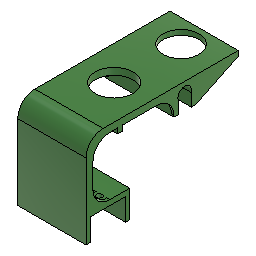
5_Assembly_Support Bat v5 (Autodesk Fusion 360 archive; units mm, degrees)
design "Support Button"
Autodesk Fusion 360 part; units mm, degrees
sketch "Sketch2" plane through (0, 0, 0) normal (1, 0, 0) x (0, 1, 0) in component "Support Batt"
  circle A0 centre (154.2359, 79.3135) radius 4
  line L0 (99.2359, 44.7135) -> (119.2359, 44.7135)
  line L1 (119.2359, 31.7135) -> (119.2359, 44.7135)
  line L2 (99.2359, 31.7135) -> (99.2359, 44.7135)
  line L3 (160.5859, 85.8135) -> (106.4359, 85.8135)
  line L4 (50.5431, 31.7135) -> (52.3447, 31.7135)
  line L5 (52.3447, 31.7135) -> (217.041, 31.7135) construction
  line L6 (96.4359, 75.8135) -> (96.4359, 31.7135)
  line L7 (96.4359, 31.7135) -> (98.9359, 31.7135)
  line L8 (98.9359, 44.7135) -> (119.5359, 44.7135)
  line L9 (119.5359, 44.7135) -> (119.5359, 31.7135)
  line L10 (98.9359, 44.7135) -> (98.9359, 31.7135)
  line L11 (119.5359, 31.7135) -> (122.0359, 31.7135)
  line L12 (154.2359, 83.3135) -> (160.5859, 83.3135) construction
  line L13 (160.5859, 85.8135) -> (160.5859, 70.8135)
  line L14 (158.0859, 70.8135) -> (160.5859, 70.8135)
  line L15 (158.0859, 78.2283) -> (158.0859, 70.8135)
  line L16 (150.3859, 78.2283) -> (150.3859, 70.8135)
  line L17 (150.3859, 70.8135) -> (147.8859, 70.8135)
  line L18 (150.3859, 70.8135) -> (158.0859, 70.8135) construction
  line L19 (154.2359, 79.3135) -> (154.2359, 70.8135) construction
  line L20 (147.8859, 70.8135) -> (147.8859, 71.8135)
  line L21 (137.8859, 81.8135) -> (110.4359, 81.8135)
  line L22 (122.0359, 31.7135) -> (122.0359, 47.7135)
  line L23 (122.0359, 47.7135) -> (110.4359, 47.7135)
  line L24 (100.4359, 57.7135) -> (100.4359, 71.8135)
  arc A1 (110.4359, 81.8135) -> (100.4359, 71.8135) centre (110.4359, 71.8135) ccw
  arc A2 (147.8859, 71.8135) -> (137.8859, 81.8135) centre (137.8859, 71.8135) ccw
  arc A3 (100.4359, 57.7135) -> (110.4359, 47.7135) centre (110.4359, 57.7135) ccw
  arc A4 (158.0859, 78.2283) -> (150.3859, 78.2283) centre (154.2359, 79.3135) ccw
  arc A5 (106.4359, 85.8135) -> (96.4359, 75.8135) centre (106.4359, 75.8135) ccw
  line L25 (114.8859, 81.8135) -> (117.8859, 81.8135)
  line L26 (117.8859, 81.8135) -> (117.8859, 78.8135)
  line L27 (117.8859, 78.8135) -> (114.8859, 78.8135)
  line L28 (114.8859, 78.8135) -> (114.8859, 81.8135)
  line L29 (160.5859, 85.8135) -> (185.5859, 85.8135)
  line L30 (185.5859, 85.8135) -> (185.5859, 82.8135)
  line L31 (185.5859, 82.8135) -> (160.5859, 82.8135)
  line L32 (160.5859, 82.8135) -> (160.5859, 85.8135)
  line L33 (160.5859, 70.8135) -> (185.5859, 82.8135)
  point P0 (96.4359, 85.8135)
  point P1 (100.4359, 81.8135)
  dimension "d2" = 0.3
  dimension "d3" = 0.3
  dimension "d4" = 2.5
  dimension "d5" = 2.5
  dimension "d6" = 2.5
  dimension "d7" = 2.5
  dimension "d8" = 8
  dimension "d9" = 15
  dimension "d10" = 7.7
  dimension "d11" = 2.5
  dimension "d12" = 4
  dimension "d13" = 4
  dimension "d14" = 3
  dimension "d15" = 10
  dimension "d68" = 10
  dimension "d69" = 3
  dimension "d70" = 3
  dimension "d71" = 30
  dimension "d80" = 25
  dimension "d81" = 3
  constraint horizontal L3
  constraint horizontal L4
  constraint parallel L4 L5
  constraint coincident L2.start L5
  constraint coincident L5 L6.end
  constraint perpendicular L5 L6
  constraint coincident L5 L7.end
  constraint perpendicular L6 L8
  constraint coincident L5 L9.end
  constraint perpendicular L8 L9
  constraint perpendicular L7 L10
  constraint coincident L0.start L8
  constraint coincident L5 L11.end
  constraint parallel L3 L12
  constraint vertical L13
  constraint horizontal L14
  constraint concentric A0 A4
  constraint coincident A0 L15.start
  constraint vertical L15
  constraint coincident A0 L16.start
  constraint vertical L16
  constraint perpendicular L16 L17
  constraint horizontal L18
  constraint coincident A0.centre L19.start
  constraint midpoint L18 L19.end
  constraint vertical L19
  constraint tangent L12 A4
  constraint perpendicular L17 L20
  constraint perpendicular L20 L21
  constraint coincident A0 L12.start
  constraint perpendicular L11 L22
  constraint perpendicular L22 L23
  constraint vertical L24
  constraint coincident P1 L21
  constraint coincident P1 L24
  constraint tangent L21 A1
  constraint tangent L24 A1
  constraint tangent L21 A2
  constraint tangent L20 A2
  constraint equal A1 A2
  constraint tangent L23 A3
  constraint tangent L24 A3
  constraint equal A1 A3
  constraint coincident P0 L6
  constraint coincident P0 L3
  constraint tangent L3 A5
  constraint tangent L6 A5
  constraint horizontal L25
  constraint vertical L26
  constraint horizontal L27
  constraint vertical L28
  constraint coincident L21 L25.start
  constraint horizontal L29
  constraint vertical L30
  constraint horizontal L31
  constraint vertical L32
  measures "d2" distance of L2.start L7.end
  measures "d3" distance of L1.start L9.end
  measures "d4" distance of L6.end L7.end
  measures "d5" distance of L9.end L11.end
  measures "d6" distance of L3 L12
  measures "d7" distance of L13.end L14.start
  measures "d8" diameter of A4
  measures "d9" distance of L3.start L13.end
  measures "d10" distance of L14.start L16.end
  measures "d11" distance of L16 L20
  measures "d12" distance of L3 L21
  measures "d13" horizontal distance of P0 P1
  measures "d14" vertical distance of L8.end L22.end
  measures "d15" radius of A1
  measures "d68" radius of A5
  measures "d69" distance of L26.end L27.end
  measures "d70" distance of L25.start L27.end
  measures "d71" horizontal distance of L17.end L26.end
  measures "d80" distance of L3.start L29.end
  measures "d81" distance of L3.start L31.end
extrude "Extrude1" add sketch "Sketch2" along normal blind 40 contours A0 L0 L3 L6 L7 L8 L9 L10 L11 L13 L14 L15 L16 L17 L20 L21 L22 L23 L24 A1 A2 A3 A4 A5 L25 L32 | L13 L29 L30 L31 L32 | L21 L25 L26 L27 L28 in component "Support Batt"
sketch "Sketch3" plane through (0, 0, 44.7135) normal (0, 0, -1) x (1, 0, 0) in component "Support Batt"
  line L0 (0, -98.9359) -> (0, -119.5359)
  line L1 (0, -119.5359) -> (40, -119.5359)
  line L2 (40, -119.5359) -> (40, -98.9359)
  line L3 (40, -98.9359) -> (0, -98.9359)
  line L4 (0, -109.2359) -> (40, -109.2359) construction
  circle A0 centre (25, -109.2359) radius 1.6
  circle A1 centre (15, -109.2359) radius 1.6
  line L5 (15, -109.2359) -> (25, -109.2359)
  line L6 (20, -109.2359) -> (20, -98.9359)
  circle A2 centre (35, -109.2359) radius 1.6
  circle A3 centre (5, -109.2359) radius 1.6
  dimension "d18" = 3.2
  dimension "d19" = 3.2
  dimension "d33" = 3.2
  dimension "d34" = 3.2
  dimension "d35" = 10
  dimension "d36" = 10
  dimension "d72" = 10
  constraint midpoint L0 L4.start
  constraint midpoint L2 L4.end
  constraint coincident L4 A0.centre
  constraint coincident L4 A1.centre
  constraint coincident A1.centre L5.start
  constraint coincident A0.centre L5.end
  constraint midpoint L5 L6.start
  constraint midpoint L3 L6.end
  constraint vertical L6
  constraint coincident L4 A2.centre
  constraint coincident L4 A3.centre
  measures "d18" diameter of A0
  measures "d19" diameter of A1
  measures "d33" diameter of A2
  measures "d34" diameter of A3
  measures "d35" distance of A1.centre A3.centre
  measures "d36" distance of A0.centre A2.centre
  measures "d72" distance of A0.centre A1.centre
extrude "Extrude2" cut sketch "Sketch3" against normal blind 17 contours A0 | A1 | A2 | A3 in component "Support Batt"
sketch "Sketch4" plane through (0, 0, 47.7135) normal (0, 0, 1) x (-1, 0, 0) in component "Support Batt"
  arc A0 (-26.0583, -110.4359) -> (-23.9417, -110.4359) centre (-25, -109.2359) ccw
  line L0 (-26.0583, -110.4359) -> (-33.9417, -110.4359)
  line L1 (-40, -110.4359) -> (-40, -122.0359)
  line L2 (-40, -122.0359) -> (0, -122.0359)
  line L3 (0, -122.0359) -> (0, -110.4359)
  line L4 (0, -110.4359) -> (-3.9417, -110.4359)
  arc A1 (-16.0583, -110.4359) -> (-13.9417, -110.4359) centre (-15, -109.2359) ccw
  line L5 (-16.0583, -110.4359) -> (-23.9417, -110.4359)
  circle A2 centre (-15, -109.2359) radius 3.25
  circle A3 centre (-25, -109.2359) radius 3.25
  arc A4 (-36.0583, -110.4359) -> (-33.9417, -110.4359) centre (-35, -109.2359) ccw
  line L6 (-36.0583, -110.4359) -> (-40, -110.4359)
  arc A5 (-6.0583, -110.4359) -> (-3.9417, -110.4359) centre (-5, -109.2359) ccw
  line L7 (-6.0583, -110.4359) -> (-13.9417, -110.4359)
  circle A6 centre (-5, -109.2359) radius 3.25
  circle A7 centre (-35, -109.2359) radius 3.25
  dimension "d22" = 6.5
  dimension "d23" = 6.5
  dimension "d37" = 6.5
  dimension "d38" = 6.5
  constraint concentric A1 A2
  constraint concentric A0 A3
  constraint concentric A5 A6
  constraint concentric A4 A7
  measures "d22" diameter of A2
  measures "d23" diameter of A3
  measures "d37" diameter of A6
  measures "d38" diameter of A7
extrude "Extrude3" cut sketch "Sketch4" along normal blind 1.0447 contours A0 L0 L5 A3 | L0 A4 L6 A7 | A1 L5 A2 L7 | L4 A5 L7 A6 picked at (-25.046, -108.9536) picked at (-35.046, -108.9536) picked at (-15.046, -108.9536) picked at (-5.046, -108.9536) in component "Support Batt"
extrude "Extrude3'" add sketch "Sketch2" along normal blind 4 contours L13 L31 L33 in component "Support Batt"
sketch "Sketch5" plane through (40, 0, 0) normal (1, 0, 0) x (0, 1, 0) in component "Support Batt"
  line L0 (158.0859, 70.8135) -> (160.5859, 70.8135)
  line L1 (160.5859, 70.8135) -> (160.5859, 82.8135)
  line L2 (160.5859, 82.8135) -> (185.5859, 82.8135)
  line L3 (185.5859, 82.8135) -> (185.5859, 85.8135)
  line L4 (185.5859, 85.8135) -> (106.4359, 85.8135)
  arc A0 (106.4359, 85.8135) -> (96.4359, 75.8135) centre (106.4359, 75.8135) ccw
  line L5 (96.4359, 75.8135) -> (96.4359, 31.7135)
  line L6 (96.4359, 31.7135) -> (98.9359, 31.7135)
  line L7 (98.9359, 31.7135) -> (98.9359, 44.7135)
  line L8 (98.9359, 44.7135) -> (119.5359, 44.7135)
  line L9 (119.5359, 44.7135) -> (119.5359, 31.7135)
  line L10 (119.5359, 31.7135) -> (122.0359, 31.7135)
  line L11 (122.0359, 31.7135) -> (122.0359, 47.7135)
  line L12 (122.0359, 47.7135) -> (110.4359, 47.7135)
  arc A1 (100.4359, 57.7135) -> (110.4359, 47.7135) centre (110.4359, 57.7135) ccw
  line L13 (100.4359, 57.7135) -> (100.4359, 71.8135)
  arc A2 (110.4359, 81.8135) -> (100.4359, 71.8135) centre (110.4359, 71.8135) ccw
  line L14 (110.4359, 81.8135) -> (114.8859, 81.8135)
  line L15 (114.8859, 81.8135) -> (114.8859, 78.8135)
  line L16 (114.8859, 78.8135) -> (117.8859, 78.8135)
  line L17 (117.8859, 78.8135) -> (117.8859, 81.8135)
  line L18 (117.8859, 81.8135) -> (137.8859, 81.8135)
  arc A3 (147.8859, 71.8135) -> (137.8859, 81.8135) centre (137.8859, 71.8135) ccw
  line L19 (147.8859, 71.8135) -> (147.8859, 70.8135)
  line L20 (147.8859, 70.8135) -> (150.3859, 70.8135)
  line L21
  arc A4 (158.0859, 78.2283) -> (150.3859, 78.2283) centre (154.2359, 79.3135) ccw
  line L22 (158.0859, 78.2283) -> (158.0859, 70.8135)
  line L23 (160.5859, 70.8135) -> (185.5859, 82.8135)
  constraint coincident L0.end L1.start
  constraint coincident L2.end L3.start
extrude "Extrude4" add sketch "Sketch5" against normal blind 4 in component "Support Batt"
sketch "Sketch4 (1)" plane through (0, 0, 81.8135) normal (0, 0, -1) x (1, 0, 0) in component "Support Batt"
  line L0 (0, -117.8859) -> (0, -137.8859)
  line L1 (0, -137.8859) -> (40, -137.8859)
  line L2 (40, -137.8859) -> (40, -117.8859)
  line L3 (40, -117.8859) -> (0, -117.8859)
  line L4 (0, -147.8859) -> (40, -147.8859)
  line L5 (40, -147.8859) -> (0, -117.8859) construction
  line L6 (0, -158.0859) -> (0, -160.5859) construction
  line L7 (0, -160.5859) -> (4, -160.5859) construction
  line L8 (4, -160.5859) -> (36, -160.5859) construction
  line L9 (36, -160.5859) -> (40, -160.5859) construction
  line L10 (40, -160.5859) -> (40, -158.0859) construction
  line L11 (40, -158.0859) -> (0, -158.0859) construction
  line L12 (0, -160.5859) -> (0, -185.5859) construction
  line L13 (0, -185.5859) -> (4, -185.5859) construction
  line L14 (4, -185.5859) -> (4, -160.5859) construction
  line L15 (4, -160.5859) -> (0, -160.5859) construction
  circle A0 centre (20, -172.0859) radius 10.5
  circle A1 centre (20, -132.8859) radius 11
  line L16 (1.5, -147.8859) -> (38.5, -147.8859)
  line L17 (38.5, -147.8859) -> (38.5, -117.8859)
  line L18 (38.5, -117.8859) -> (1.5, -117.8859)
  line L19 (1.5, -117.8859) -> (1.5, -147.8859)
  line L20 (1.5, -147.8859) -> (38.5, -117.8859) construction
  line L21 (38.5, -147.8859) -> (1.5, -117.8859) construction
  line L22 (20, -158.0859) -> (20, -172.0859)
  point P0 (20, -132.8859)
  dimension "d88" = 21
  dimension "d89" = 22
  dimension "d90" = 37
  dimension "d91" = 30
  dimension "d96" = 14
  constraint coincident L4.end L5.start
  constraint coincident L0.start L3.end
  constraint midpoint L5 P0
  constraint horizontal L16
  constraint perpendicular L16 L17
  constraint parallel L16 L18
  constraint parallel L17 L19
  constraint coincident L20 P0
  constraint coincident L21 P0
  constraint coincident P0 A1.centre
  constraint midpoint L11 L22.start
  constraint coincident A0.centre L22.end
  constraint perpendicular L8 L22
  measures "d88" diameter of A0
  measures "d89" diameter of A1
  measures "d90" distance of L17.end L18.end
  measures "d91" distance of L16.end L17.end
  measures "d96" distance of L22.start A0.centre
extrude "Extrude5" cut sketch "Sketch4 (1)" against normal blind 11 contours L1 A1 | L1 A1 | A0 in component "Support Batt"
extrude "Extrude6" cut sketch "Sketch4 (1)" along normal blind 17 contours L1 L4 A1 L16 L17 L19 | L1 A1 picked at (22.1414, -140.7456) in component "Support Batt"
component "Support Batt" placed x (1, 0, 0) y (0, 1, 0) z (0, 0, 1) at (0, 0, 0)
named bodies: "Support_Button"

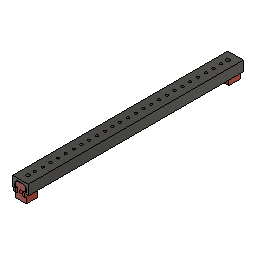
design "Support CI"
Autodesk Fusion 360 part; units mm, degrees
sketch "Sketch1" plane through (0, 0, 0) normal (0, 0, 1) x (1, 0, 0) in component "Support Electo"
  line L0 (138.5, -10) -> (-138.5, -10)
  line L1 (-138.5, -10) -> (-138.5, 10)
  line L2 (-138.5, 10) -> (138.5, 10)
  line L3 (138.5, 10) -> (138.5, -10)
  line L4 (138.5, -10) -> (-138.5, 10) construction
  line L5 (-138.5, -10) -> (138.5, 10) construction
  line L6 (138.5, -10) -> (138.5, 10)
  circle A0 centre (0, 0) radius 1.6
  circle A1 centre (-120, 0) radius 1.6
  circle A2 centre (-110, 0) radius 1.6
  circle A3 centre (-100, 0) radius 1.6
  circle A4 centre (-90, 0) radius 1.6
  circle A5 centre (-80, 0) radius 1.6
  circle A6 centre (-70, 0) radius 1.6
  circle A7 centre (-60, 0) radius 1.6
  circle A8 centre (-50, 0) radius 1.6
  circle A9 centre (-40, 0) radius 1.6
  circle A10 centre (-30, 0) radius 1.6
  circle A11 centre (-20, 0) radius 1.6
  circle A12 centre (-10, 0) radius 1.6
  circle A13 centre (10, 0) radius 1.6
  circle A14 centre (20, 0) radius 1.6
  circle A15 centre (30, 0) radius 1.6
  circle A16 centre (40, 0) radius 1.6
  circle A17 centre (50, 0) radius 1.6
  circle A18 centre (60, 0) radius 1.6
  circle A19 centre (70, 0) radius 1.6
  circle A20 centre (80, 0) radius 1.6
  circle A21 centre (90, 0) radius 1.6
  circle A22 centre (100, 0) radius 1.6
  circle A23 centre (110, 0) radius 1.6
  circle A24 centre (120, 0) radius 1.6
  line L7 (-138.5, 10) -> (138.5, 10)
  line L8 (138.5, 10) -> (138.5, 7)
  line L9 (138.5, 7) -> (-138.5, 7)
  line L10 (-138.5, 7) -> (-138.5, 10)
  line L11 (-138.5, -7) -> (138.5, -7)
  line L12 (138.5, -7) -> (138.5, -10)
  line L13 (138.5, -10) -> (-138.5, -10)
  line L14 (-138.5, -10) -> (-138.5, -7)
  line L15 (-138.5, -10) -> (-138.5, -7)
  line L16 (-138.5, 7) -> (-138.5, 10)
  circle A25 centre (-128.5, 0) radius 2.25
  circle A26 centre (128.5, 0) radius 2.25
  line L17 (-138.5, 0) -> (138.5, 0) construction
  dimension "d171" = 277
  dimension "d172" = 20
  dimension "d174" = 20
  dimension "d176" = 20
  dimension "d189" = 3.2
  dimension "d192" = 10
  dimension "d193" = 0
  dimension "d194" = 3
  dimension "d195" = 3
  dimension "d225" = 4.5
  dimension "d226" = 10
  dimension "d227" = 4.5
  dimension "d228" = 10
  constraint horizontal L0
  constraint perpendicular L0 L1
  constraint parallel L0 L2
  constraint parallel L1 L3
  constraint coincident L4 A0.centre
  constraint coincident L5 A0.centre
  constraint coincident A0.centre origin
  constraint vertical L15
  constraint vertical L6
  constraint horizontal L7
  constraint vertical L8
  constraint horizontal L9
  constraint vertical L10
  constraint coincident L3 L8.end
  constraint horizontal L11
  constraint vertical L12
  constraint horizontal L13
  constraint vertical L14
  constraint collinear L15 L16
  constraint midpoint L1 L17.start
  constraint midpoint L6 L17.end
  constraint coincident A26.centre L17
  constraint coincident A25.centre L17
  measures "d171" distance of L1.end L2.end
  measures "d172" distance of L0.end L1.end
  measures "d174" distance of L1.end L0.end
  measures "d176" distance of L2.end L0.start
  measures "d189" diameter of A0
  measures "d194" distance of L1.end L9.end
  measures "d195" distance of L11.start L0.end
  measures "d225" diameter of A25
  measures "d226" distance of L1 A25.centre
  measures "d227" diameter of A26
  measures "d228" distance of L6 A26.centre
extrude "Extrude6" add sketch "Sketch1" along normal blind 3 makes body 1 in component "Support Electo"
extrude "Extrude7" add sketch "Sketch1" against normal blind 10 contours L0 L1 L3 L6 L11 L12 L13 L14 L15 | L1 L2 L3 L6 L7 L8 L9 L10 L16 bodies 1 in component "Support Electo"
fillet "Fillet2" radius 4 2 edges at (0, 7, 0) (0, -7, 0) on bodies 1 in component "Support Electo"
sketch "Sketch1 (2)" plane through (0, 4.3249, 0) normal (0, -1, 0) x (1, 0, 0) in component "Equerre"
  line L0 (266.4871, 11.1429) -> (266.4871, 24.1429)
  line L1 (266.4871, 24.1429) -> (246.4871, 24.1429)
  line L2 (246.4871, 24.1429) -> (246.4871, 11.1429)
  line L3 (246.4871, 11.1429) -> (249.4871, 11.1429)
  line L4 (249.4871, 11.1429) -> (249.4871, 17.1429)
  arc A0 (253.4871, 21.1429) -> (249.4871, 17.1429) centre (253.4871, 17.1429) ccw
  line L5 (253.4871, 21.1429) -> (259.4871, 21.1429)
  arc A1 (263.4871, 17.1429) -> (259.4871, 21.1429) centre (259.4871, 17.1429) ccw
  line L6 (263.4871, 17.1429) -> (263.4871, 11.1429)
  line L7 (263.4871, 11.1429) -> (266.4871, 11.1429)
  arc A2 (263.4871, 17.1429) -> (259.4871, 21.1429) centre (259.4871, 17.1429) ccw
  line L8 (263.4871, 17.1429) -> (263.4871, 11.1429)
  line L9 (259.4871, 21.1429) -> (253.4871, 21.1429)
  arc A3 (253.4871, 21.1429) -> (249.4871, 17.1429) centre (253.4871, 17.1429) ccw
  line L10 (249.4871, 17.1429) -> (249.4871, 11.1429)
  line L11 (263.3871, 17.1429) -> (263.3871, 5.9705)
  line L12 (249.5871, 17.1429) -> (249.5871, 5.9705)
  arc A4 (253.4871, 21.0429) -> (249.5871, 17.1429) centre (253.4871, 17.1429) ccw
  line L13 (259.4871, 21.0429) -> (253.4871, 21.0429)
  arc A5 (263.3871, 17.1429) -> (259.4871, 21.0429) centre (259.4871, 17.1429) ccw
  line L14 (263.3871, 5.9705) -> (263.3871, 1.0429)
  line L15 (263.3871, 1.0429) -> (249.5871, 1.0429)
  line L16 (249.5871, 1.0429) -> (249.5871, 5.9705)
  line L17 (249.5871, 10.9429) -> (249.5871, 11.1429)
  line L18 (263.3871, 11.1429) -> (263.3871, 10.9429)
  line L19 (249.4871, 11.1429) -> (249.5871, 11.1429)
  circle A6 centre (256.4871, 11.0429) radius 2.1
  line L20 (249.5871, 11.0429) -> (263.3871, 11.0429) construction
  line L21 (263.3871, 8.0429) -> (249.5871, 8.0429)
  line L22 (249.5871, 8.0429) -> (249.5871, 14.0429)
  line L23 (249.5871, 14.0429) -> (263.3871, 14.0429)
  line L24 (263.3871, 14.0429) -> (263.3871, 8.0429)
  line L25 (263.3871, 8.0429) -> (249.5871, 14.0429) construction
  line L26 (249.5871, 8.0429) -> (263.3871, 14.0429) construction
  line L27 (260.9871, 8.0429) -> (251.9871, 8.0429)
  line L28 (251.9871, 8.0429) -> (251.9871, 14.0429)
  line L29 (251.9871, 14.0429) -> (260.9871, 14.0429)
  line L30 (260.9871, 14.0429) -> (260.9871, 8.0429)
  line L31 (260.9871, 8.0429) -> (251.9871, 14.0429) construction
  line L32 (251.9871, 8.0429) -> (260.9871, 14.0429) construction
  point P0 (256.4871, 11.0429)
  point P1 (256.4871, 11.0429)
  point P2 (256.4871, 11.0429)
  dimension "d268" = 4.2
  dimension "d273" = 20
  dimension "d274" = 0.1
  dimension "d275" = 10
  dimension "d276" = 6
  dimension "d282" = 9
  constraint coincident L3.end L4.start
  constraint vertical L14
  constraint horizontal L15
  constraint vertical L16
  constraint coincident L11.end L14.start
  constraint parallel L17 L18
  constraint coincident L14 L18.start
  constraint parallel L8 L11
  constraint parallel L10 L12
  constraint concentric A3 A4
  constraint parallel L9 L13
  constraint concentric A2 A5
  constraint tangent L13 A5
  constraint tangent L11 A5
  constraint tangent A4 L13
  constraint tangent L12 A4
  constraint coincident P2 P1
  constraint coincident L12 L20.start
  constraint coincident L11 L20.end
  constraint perpendicular L11 L20
  constraint coincident P2 L20
  constraint midpoint P2 L20
  constraint horizontal L21
  constraint perpendicular L21 L22
  constraint parallel L21 L23
  constraint parallel L22 L24
  constraint coincident L11 L21.start
  constraint coincident L25 P2
  constraint coincident L26 P2
  constraint horizontal L27
  constraint perpendicular L27 L28
  constraint parallel L27 L29
  constraint parallel L28 L30
  constraint coincident L31 P2
  constraint coincident L32 P2
  constraint coincident L21 L27.start
  measures "d268" diameter of A6
  measures "d273" distance of L13 L15
  measures "d274" distance of L4 L12
  measures "d275" distance of L15 L20
  measures "d276" distance of L21 L23
  measures "d282" distance of L28.end L29.end
extrude "Extrude1" add sketch "Sketch1 (2)" against normal blind 15 separate body contours L11 L12 A4 L13 A5 L23 L29 | L11 L18 L21 L23 L24 L30 | L21 L23 L27 L28 L29 L30 | L12 L17 L21 L22 L23 L28 | L11 L12 L14 L15 L16 L21 L27 makes body 2 in component "Equerre"
extrude "Extrude3" add sketch "Sketch1 (2)" along normal blind 2 contours L11 L18 L21 L23 L24 L30 | L12 L17 L21 L22 L23 L28 bodies 2 in component "Equerre"
sketch "Sketch2" plane through (0, 0, 21.1429) normal (0, 0, -1) x (1, 0, 0) in component "Equerre"
  line L0 (259.4871, -281.3249) -> (259.4871, -4.3249)
  line L1 (259.4871, -4.3249) -> (253.4871, -4.3249)
  line L2 (253.4871, -4.3249) -> (253.4871, -281.3249)
  line L3 (253.4871, -281.3249) -> (259.4871, -281.3249)
  circle A0 centre (256.4871, -142.8249) radius 1.6
  circle A1 centre (256.4871, -22.8249) radius 1.6
  circle A2 centre (256.4871, -32.8249) radius 1.6
  circle A3 centre (256.4871, -42.8249) radius 1.6
  circle A4 centre (256.4871, -52.8249) radius 1.6
  circle A5 centre (256.4871, -62.8249) radius 1.6
  circle A6 centre (256.4871, -72.8249) radius 1.6
  circle A7 centre (256.4871, -82.8249) radius 1.6
  circle A8 centre (256.4871, -92.8249) radius 1.6
  circle A9 centre (256.4871, -102.8249) radius 1.6
  circle A10 centre (256.4871, -112.8249) radius 1.6
  circle A11 centre (256.4871, -132.8249) radius 1.6
  circle A12 centre (256.4871, -122.8249) radius 1.6
  circle A13 centre (256.4871, -212.8249) radius 1.6
  circle A14 centre (256.4871, -202.8249) radius 1.6
  circle A15 centre (256.4871, -192.8249) radius 1.6
  circle A16 centre (256.4871, -182.8249) radius 1.6
  circle A17 centre (256.4871, -172.8249) radius 1.6
  circle A18 centre (256.4871, -162.8249) radius 1.6
  circle A19 centre (256.4871, -152.8249) radius 1.6
  circle A20 centre (256.4871, -271.3249) radius 2.25
  circle A21 centre (256.4871, -222.8249) radius 1.6
  circle A22 centre (256.4871, -232.8249) radius 1.6
  circle A23 centre (256.4871, -242.8249) radius 1.6
  circle A24 centre (256.4871, -252.8249) radius 1.6
  circle A25 centre (256.4871, -262.8249) radius 1.6
  circle A26 centre (256.4871, -14.4249) radius 0.75
  line L4 (256.4871, -4.3249) -> (256.4871, -14.4249) construction
  dimension "d277" = 1.5
  dimension "d279" = 10.1
  constraint midpoint L1 L4.start
  constraint coincident A26.centre L4.end
  constraint perpendicular L1 L4
  measures "d277" diameter of A26
  measures "d279" distance of L1 A26.centre
extrude "Extrude2" cut sketch "Sketch2" along normal blind 11 contours A26 bodies 2 in component "Equerre"
sketch "Sketch3" plane through (0, 19.3249, 0) normal (0, 1, 0) x (-1, 0, 0) in component "Equerre"
  circle A0 centre (-256.4871, 11.0429) radius 2.1
  line L0 (-263.3871, 17.1429) -> (-263.3871, 1.0429)
  line L1 (-263.3871, 1.0429) -> (-249.5871, 1.0429)
  line L2 (-249.5871, 1.0429) -> (-249.5871, 17.1429)
  arc A1 (-249.5871, 17.1429) -> (-253.4871, 21.0429) centre (-253.4871, 17.1429) ccw
  line L3 (-253.4871, 21.0429) -> (-259.4871, 21.0429)
  arc A2 (-259.4871, 21.0429) -> (-263.3871, 17.1429) centre (-259.4871, 17.1429) ccw
  circle A3 centre (-256.4871, 11.0429) radius 5
  dimension "d269" = 10
  constraint concentric A0 A3
  measures "d269" diameter of A3
extrude "Extrude4" cut sketch "Sketch3" against normal blind 8 contours A3 bodies 2 in component "Equerre"
chamfer "Chamfer1" distance 1.5 angle 45 2 edges at (262.1871, 2.3249, 8.0429) (250.7871, 2.3249, 8.0429) on bodies 2 in component "Equerre"
component "Support Electo" placed x (0, 1, 0) y (-1, 0, 0) z (0, 0, 1) at (230.1725, 147.8044, 52.437)
component "Equerre" placed x (1, 0, 0) y (0, 1, 0) z (0, 0, 1) at (-25.5646, 4.8794, 31.394)
component "Equerre" placed x (-1, 0, 0) y (0, -1, 0) z (0, 0, 1) at (485.9095, 290.7293, 31.394)
named bodies: "Equerre_Support_CI"

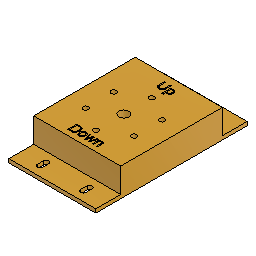
design "Support Suspension - IN"
Autodesk Fusion 360 part; units mm, degrees
sketch "Sketch1" plane through (0, 0, 0) normal (0, 0, 1) x (1, 0, 0)
  line L0 (-35, 60.9) -> (35, 60.9)
  line L1 (35, 60.9) -> (35, -60.9)
  line L2 (35, -60.9) -> (-35, -60.9)
  line L3 (-35, -60.9) -> (-35, 60.9)
  line L4 (-35, 60.9) -> (35, -60.9) construction
  line L5 (35, 60.9) -> (-35, -60.9) construction
  line L6 (35, -40.9) -> (-35, -40.9)
  line L7 (-35, -40.9) -> (-35, 40.9)
  line L8 (-35, 40.9) -> (35, 40.9)
  line L9 (35, 40.9) -> (35, -40.9)
  line L10 (35, -40.9) -> (-35, 40.9) construction
  line L11 (-35, -40.9) -> (35, 40.9) construction
  line L12 (-35, -3.3) -> (35, -3.3) construction
  circle A0 centre (0, -3.3) radius 4
  circle A1 centre (0, -3.3) radius 22.5 construction
  line L13 (0, 0) -> (0, 2.2401)
  line L14 (0, 2.2401) -> (0, 60.9) construction
  circle A2 centre (0, 19.2) radius 2.1
  circle A3 centre (-19.4856, 7.95) radius 2.1
  circle A4 centre (-19.4856, -14.55) radius 2.1
  circle A5 centre (0, -25.8) radius 2.1
  circle A6 centre (19.4856, -14.55) radius 2.1
  circle A7 centre (19.4856, 7.95) radius 2.1
  line L15 (-35, 60.9) -> (35, 40.9) construction
  line L16 (0, 50.9) -> (-35, 50.9) construction
  line L17 (0, 50.9) -> (35, 50.9) construction
  line L18 (-19.6, 53.4) -> (-19.6, 48.4)
  arc A8 (-19.6, 48.4) -> (-15.4, 48.4) centre (-17.5, 48.4) ccw
  line L19 (-15.4, 48.4) -> (-15.4, 53.4)
  arc A9 (-15.4, 53.4) -> (-19.6, 53.4) centre (-17.5, 53.4) ccw
  line L20 (-17.5, 53.4) -> (-17.5, 48.4) construction
  arc A10 (19.6, 53.4) -> (15.4, 53.4) centre (17.5, 53.4) ccw
  line L21 (19.6, 53.4) -> (19.6, 48.4)
  arc A11 (15.4, 48.4) -> (19.6, 48.4) centre (17.5, 48.4) ccw
  line L22 (15.4, 48.4) -> (15.4, 53.4)
  line L23 (-35, 0) -> (35, 0) construction
  arc A12 (15.4, -53.4) -> (19.6, -53.4) centre (17.5, -53.4) ccw
  arc A13 (-15.4, -48.4) -> (-19.6, -48.4) centre (-17.5, -48.4) ccw
  arc A14 (-19.6, -53.4) -> (-15.4, -53.4) centre (-17.5, -53.4) ccw
  arc A15 (19.6, -48.4) -> (15.4, -48.4) centre (17.5, -48.4) ccw
  line L24 (-17.5, -53.4) -> (-17.5, -48.4) construction
  line L25 (-15.4, -48.4) -> (-15.4, -53.4)
  line L26 (19.6, -53.4) -> (19.6, -48.4)
  line L27 (15.4, -48.4) -> (15.4, -53.4)
  line L28 (-19.6, -53.4) -> (-19.6, -48.4)
  line L29 (0, -50.9) -> (-35, -50.9) construction
  point P0 (-17.5, 50.9)
  point P1 (-17.5, -50.9)
  dimension "d1" = 121.8
  dimension "d2" = 70
  dimension "d3" = 81.8
  dimension "d4" = 44.2
  dimension "d5" = 38.6
  dimension "d6" = 8
  dimension "d7" = 45
  dimension "d8" = 4.2
  dimension "d10" = 360
  dimension "d13" = 4.2
  dimension "d14" = 5
  dimension "d19" = 3.3
  constraint perpendicular L0 L1
  constraint parallel L0 L2
  constraint parallel L1 L3
  constraint horizontal L0
  constraint coincident L4 L13.start
  constraint coincident L5 L13.start
  constraint coincident L13.start origin
  constraint perpendicular L6 L7
  constraint parallel L6 L8
  constraint parallel L7 L9
  constraint horizontal L6
  constraint coincident L1 L6.start
  constraint coincident L10 L13.start
  constraint coincident L11 L13.start
  constraint coincident L7 L12.start
  constraint coincident L9 L12.end
  constraint perpendicular L7 L12
  constraint midpoint L12 A0.centre
  constraint concentric A0 A1
  constraint vertical L13
  constraint midpoint L0 L14.end
  constraint coincident A1 A2.centre
  constraint coincident L14 A2.centre
  constraint midpoint L15 L16.start
  constraint coincident L3 L16.end
  constraint perpendicular L3 L16
  constraint coincident L1 L17.end
  constraint perpendicular L1 L17
  constraint tangent L18 A8
  constraint tangent A8 L19
  constraint parallel L18 L19
  constraint tangent L19 A9
  constraint tangent L18 A9
  constraint perpendicular L16 L20
  constraint midpoint L16 P0
  constraint midpoint L20 P0
  constraint symmetric L14 L18.start A10.start
  constraint symmetric L14 L18.end L21.end
  constraint symmetric L14 A8.end A11.start
  constraint symmetric L14 L19.end A10.end
  constraint symmetric L14 A8 A11
  constraint symmetric L14 A9 A10
  constraint midpoint L9 L23.end
  constraint perpendicular L9 L23
  constraint symmetric L16.start L23 L29.start
  constraint symmetric L16.end L23 L29.end
  constraint symmetric L18.start L23 A14.start
  constraint symmetric L18.end L23 A13.end
  constraint symmetric A8.end L23 A13.start
  constraint symmetric L19.end L23 A14.end
  constraint symmetric A8 L23 A13
  constraint symmetric A9 L23 A14
  constraint symmetric P0 L23 P1
  constraint symmetric A10.end L23 A12.start
  constraint symmetric A10.start L23 A12.end
  constraint symmetric A10 L23 A12
  constraint symmetric L21.end L23 A15.start
  constraint symmetric A11.start L23 A15.end
  constraint symmetric A11 L23 A15
  measures "d1" distance of L0.start L2.end
  measures "d2" distance of L0.start L0.end
  measures "d3" distance of L6.end L7.end
  measures "d4" distance of L8 L12
  measures "d6" diameter of A0
  measures "d7" diameter of A1 L0.start
  measures "d8" diameter of A2
  measures "d13" diameter of A8
  measures "d14" distance of A9.centre A8.centre
  measures "d19" distance of L13.start A0.centre
extrude "Extrude1" add sketch "Sketch1" along normal blind 19.8 contours L1 L3 L6 L7 L8 L9
extrude "Extrude2" add sketch "Sketch1" against normal blind 3
sketch "Sketch2" plane through (0, 0, 19.8) normal (0, 0, 1) x (-1, 0, 0)
  circle A0 centre (-19.4856, -7.95) radius 2.1
  circle A1 centre (-19.4856, 14.55) radius 2.1
  circle A2 centre (0, 25.8) radius 2.1
  circle A3 centre (19.4856, 14.55) radius 2.1
  circle A4 centre (19.4856, -7.95) radius 2.1
  circle A5 centre (0, -19.2) radius 2.1
  circle A6 centre (0, 3.3) radius 4
  line L0 (-35, -40.9) -> (35, -40.9)
  line L1 (35, -40.9) -> (35, 40.9)
  line L2 (35, 40.9) -> (-35, 40.9)
  line L3 (-35, 40.9) -> (-35, -40.9)
  line L4 (6.2801, -26.4921) -> (-5.3166, -26.4921) construction
  line L5 (-5.3166, -26.4921) -> (-5.3166, -36.4921) construction
  line L6 (-5.3166, -36.4921) -> (6.2801, -36.4921) construction
  line L7 (6.2801, -36.4921) -> (6.2801, -26.4921) construction
  line L8 (11.9175, 36.5887) -> (-12.1889, 36.5887) construction
  line L9 (-12.1889, 36.5887) -> (-12.1889, 26.5887) construction
  line L10 (-12.1889, 26.5887) -> (11.9175, 26.5887) construction
  line L11 (11.9175, 26.5887) -> (11.9175, 36.5887) construction
  text T0 "Up" font "Arial" height 10 align ink ink in box 0 x 0 at (6.2801, -26.4921) x (-1, 0) y (0, -1) spacing 1 kerned height is em
  text T1 "Down" font "Arial" height 10 align ink ink in box 0 x 0 at (11.9175, 36.5887) x (-1, 0) y (0, -1) spacing 1 kerned height is em
  constraint perpendicular L4 L5
  constraint parallel L4 L6
  constraint parallel L5 L7
  constraint perpendicular L8 L9
  constraint parallel L8 L10
  constraint parallel L9 L11
extrude "Extrude3" cut sketch "Sketch2" against normal blind 1 text T1 T0
named bodies: "Support Suspension"
